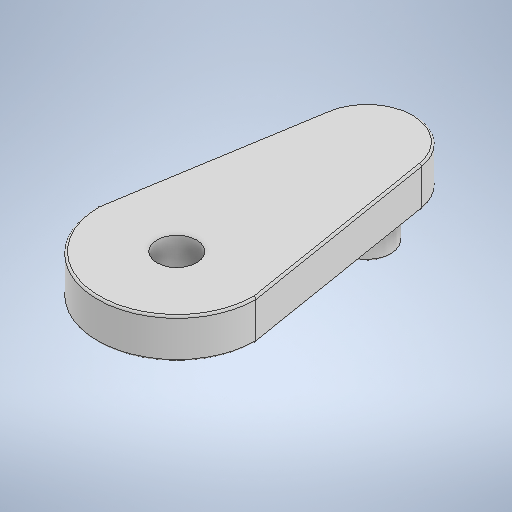
# Autodesk Inventor part: 201 part 2
Saved by Autodesk Inventor 2025.1 (Build 291241000, 241)
## iProperties
Created: 2024-09-02
Part Number: 201 part 2
Material: Generisch
Document SubType Name: Modeling
Designer: ffogue
Density: 1 g/cm^3
Appearance: Vorgabe
Author: ffogue
Autodesk Inventor part; units mm, degrees
ref_plane "YZ Plane" through (0, 0, 0) normal (1, 0, 0) x (0, 1, 0)
ref_plane "XZ Plane" through (0, 0, 0) normal (0, 1, 0) x (-1, 0, 0)
ref_plane "XY Plane" through (0, 0, 0) normal (0, 0, 1) x (1, 0, 0)
sketch "Sketch1" plane through (0, 0, 0) normal (0, 0, 1) x (1, 0, 0)
  line L0 (-10, 0) -> (10, 0) construction
  arc A0 (-10, 0) -> (10, 0) centre (0, 0) ccw
  line L1 (-10, 0) -> (-5.9215, 24.9673)
  arc A1 (5.9215, 24.9673) -> (-5.9215, 24.9673) centre (0, 24) ccw
  line L2 (5.9215, 24.9673) -> (10, 0)
  line L3 (0, 0) -> (0, 15.7423) construction
  dimension "d0" = 24
  dimension "d1" = 6
  dimension "d2" = 10
  constraints: 8 end point, 4 point on circle, 2 centre point, 2 midpoint, 2 tangent, 1 coincident, 1 horizontal, 1 vertical, 1 vertical alignment
  measures "d0" distance of point (0, 0) A1.centre
  measures "d1" radius of A1
  measures "d2" radius of A0
extrude "Extrusion1" add sketch "Sketch1" against normal blind 5
sketch "Sketch2" plane through (0, 0, 0) normal (0, 0, 1) x (1, 0, 0)
  circle A0 centre (0, 24) radius 3
  arc A1 (5.9215, 24.9673) -> (-5.9215, 24.9673) centre (0, 24) ccw projected
  point P0 (0, 0)
  dimension "d5" = 6
  constraints: 1 centre point, 1 concentric
  measures "d5" diameter of A0
extrude "Extrusion2" add sketch "Sketch2" against normal blind 11
sketch "Sketch3" plane through (0, 0, 0) normal (0, 0, 1) x (1, 0, 0)
  circle A0 centre (0, 0) radius 2.5
  dimension "d14" = 5
  constraints: 1 centre point, 1 coincident
  measures "d14" diameter of A0
extrude "Extrusion3" cut sketch "Sketch3" against normal up to surface (5 mm away)
fillet "Fillet1" radius 0.25 9 edges at (-3, 24, -11) (0, 30, -5) (-7.9608, 12.4836, -5) (7.9608, 12.4836, -5) (0, -10, -5) (0, -10, 0) (0, 30, 0) (-7.9608, 12.4836, 0) (7.9608, 12.4836, 0)
body "Solid1"
